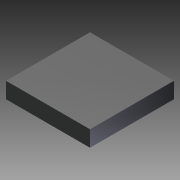
# Autodesk Inventor part: UB216KKW015C-NR
Saved by Autodesk Inventor 2015 SP1 (Build 190203100, 203)
## iProperties
Category: Electrical
Company: Autodesk Inc.
Created: 2014-12-16
Part Number: UB216KKW015C-NR
Catalog Web Link: http://www.nkkswitches.com/
Description: PC and Snap-in Mount Non-Illuminated Pushbuttons_ni_diffuser_cap-Non-Illuminated Pushbuttons - Series UB2
Vendor: NKK Switches
Document SubType Name: Modeling
Designer: Autodesk Inc.
Manufacturer: NKKSWITCHES
Mass: 0.389193 g
Surface Area: 4.4516 cm^2
Volume: 0.389193 cm^3
Density: 1 g/cm^3
Material: Generic
Appearance: PSOLRGB-192-192-192
Title: UB2KK5Cni_d_cap
Author: Autodesk Inc.
Comments: Non-Illuminated Pushbuttons - Series UB2
Autodesk Inventor part; units mm, degrees
sketch "Sketch_3" plane through (0, 0, 0) normal (0, 1, 0) x (-1, 0, 0)
  line L0 (6.35, 6.35) -> (-6.35, 6.35)
  line L1 (-6.35, 6.35) -> (-6.35, -6.35)
  line L2 (-6.35, -6.35) -> (6.35, -6.35)
  line L3 (6.35, -6.35) -> (6.35, 6.35)
  constraints: 8 end point
extrude "Extrusion1" add sketch "Sketch_3" against normal blind 2.413
ref_plane "diffuser_to_body_XY" through (0, 0, 0) normal (0, 1, 0) x (1, 0, 0)
ref_plane "diffuser_to_body_YZ" through (0, 0, 0) normal (1, 0, 0) x (0, 0, -1)
ref_plane "diffuser_to_body_ZX" through (0, 0, 0) normal (0, 0, -1) x (0, 1, 0)
ref_plane "lens2_to_body_XY" through (0, 0, 0) normal (0, 1, 0) x (1, 0, 0)
ref_plane "lens2_to_body_YZ" through (0, 0, 0) normal (1, 0, 0) x (0, 0, -1)
ref_plane "lens2_to_body_ZX" through (0, 0, 0) normal (0, 0, -1) x (0, 1, 0)
body "Solid1"
